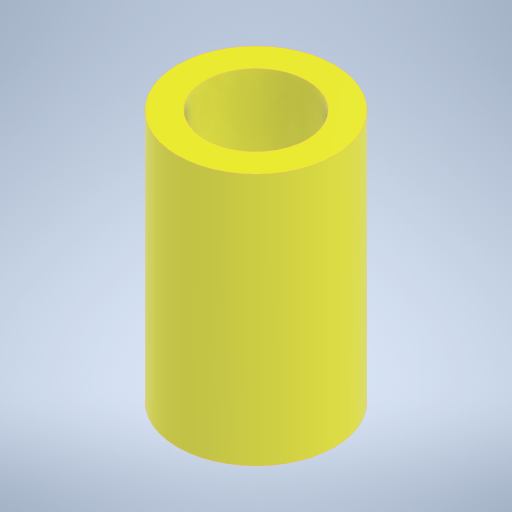
# Autodesk Inventor part: pneu
Saved by Autodesk Inventor 2023 (Build 270158000, 158)
## iProperties
Created: 2023-08-08
Part Number: pneu
Material: Resina fenólica
Document SubType Name: Modeling
Designer: azeve
Density: 1.38 g/cm^3
Appearance: Suave - Laranja claro
Author: azeve
Autodesk Inventor part; units mm, degrees
ref_plane "YZ Plane" through (0, 0, 0) normal (1, 0, 0) x (0, 1, 0)
ref_plane "XZ Plane" through (0, 0, 0) normal (0, 1, 0) x (-1, 0, 0)
ref_plane "XY Plane" through (0, 0, 0) normal (0, 0, 1) x (1, 0, 0)
sketch "Esboço1" plane through (0, 0, 0) normal (0, 0, 1) x (1, 0, 0)
  line L0 (0, 0) -> (0, 75.9)
  line L1 (15.0065, 48.298) -> (15.0065, 0)
  line L2 (15.0065, 0) -> (9.738, 0)
  line L3 (9.738, 2) -> (9.738, 48.298)
  line L4 (9.738, 2) -> (9.738, 0)
  line L5 (9.738, 48.298) -> (15.0065, 48.298)
  dimension "d0" = 75.9
  dimension "d10" = 48.298
  constraints: 12 end point, 2 vertical, 1 horizontal, 1 perpendicular, 1 point on line
  measures "d0" distance of L0.start L0.end
  measures "d10" distance of L1.end L1.start
revolve "Revolução1" add sketch "Esboço1" angle 360 about axis through (0, 0, 0) along (0, 1, 0)
